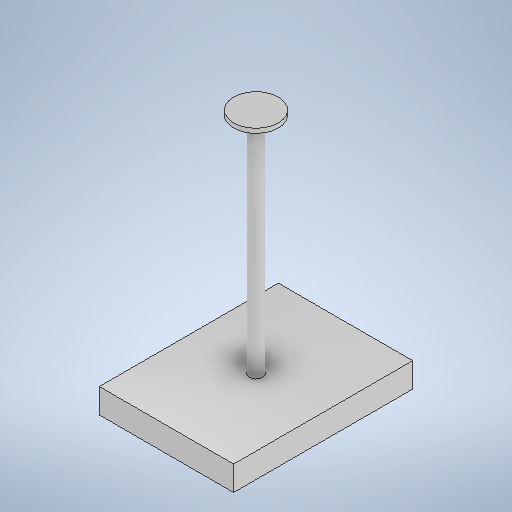
# Autodesk Inventor part: Corte
Saved by Autodesk Inventor 2025.2 (Build 292293000, 293)
## iProperties
Created: 2025-02-05
Part Number: Corte
Material: Generic
Document SubType Name: Modeling
Designer: Proyectos
Density: 1 g/cm^3
Appearance: Default
Author: Proyectos
Autodesk Inventor part; units mm, degrees
ref_plane "YZ Plane" through (0, 0, 0) normal (1, 0, 0) x (0, 1, 0)
ref_plane "XZ Plane" through (0, 0, 0) normal (0, 1, 0) x (-1, 0, 0)
ref_plane "XY Plane" through (0, 0, 0) normal (0, 0, 1) x (1, 0, 0)
sketch "Sketch1" plane through (0, 0, 0) normal (0, 1, 0) x (-1, 0, 0)
  line L0 (0, 0) -> (600, 0)
  line L1 (600, 0) -> (600, -800)
  line L2 (600, -800) -> (0, -800)
  line L3 (0, -800) -> (0, 0)
  line L4 (0, 0) -> (50, 0)
  line L5 (50, 0) -> (50, -50)
  line L6 (50, -50) -> (0, -50)
  line L7 (0, -50) -> (0, 0)
  line L8 (600, -800) -> (550, -800)
  line L9 (550, -800) -> (550, -750)
  line L10 (550, -750) -> (600, -750)
  line L11 (600, -750) -> (600, -800)
  line L12 (50, -50) -> (550, -50)
  line L13 (550, -50) -> (550, -750)
  line L14 (550, -750) -> (50, -750)
  line L15 (50, -750) -> (50, -50)
  dimension "d0" = 800
  dimension "d1" = 600
  dimension "d2" = 50
  dimension "d3" = 50
  dimension "d4" = 50
  dimension "d5" = 50
  constraints: 32 end point, 8 parallel, 4 horizontal, 4 perpendicular
  measures "d0" distance of L0.end L1.end
  measures "d1" distance of L1.end L2.end
  measures "d2" distance of L5.end L6.end
  measures "d3" distance of L4.end L5.end
  measures "d4" distance of L9.end L10.end
  measures "d5" distance of L8.end L9.end
extrude "Extrusion1" add sketch "Sketch1" along normal blind 100 contours L0 L5 L6 L3 | L0 L1 L10 L13 L12 L5 | L6 L15 L14 L9 L2 L3 | L1 L2 L9 L10
sketch "Sketch2" plane through (0, 100, 0) normal (0, 1, 0) x (1, 0, 0)
  line L0 (-600, 800) -> (-600, 0) projected
  line L1 (0, 0) -> (0, 800) projected
  line L2 (-600, 0) -> (0, 0)
  line L3 (0, 0) -> (0, 800)
  line L4 (0, 800) -> (-600, 800)
  line L5 (-600, 800) -> (-600, 0)
  circle A0 centre (-300, 400) radius 25
  dimension "d8" = 50
  constraints: 8 end point, 2 parallel, 1 centre point, 1 horizontal, 1 perpendicular
  measures "d8" diameter of A0
extrude "Extrusion2" add sketch "Sketch2" along normal blind 10 contours L4 L1 L2 L0 | A0
sketch "Sketch3" plane through (0, 110, 0) normal (0, 1, 0) x (1, 0, 0)
  line L0 (0, 0) -> (0, 800) projected
  line L1 (0, 800) -> (-600, 800) projected
  line L2 (-600, 800) -> (-600, 0) projected
  line L3 (-600, 0) -> (0, 0) projected
  circle A0 centre (-300, 400) radius 30
  dimension "d11" = 60
  constraints: 1 centre point
  measures "d11" diameter of A0
extrude "Extrusion3" add sketch "Sketch3" along normal blind 1000 contours A0
sketch "Sketch4" plane through (-300, 1110, -400) normal (0, 1, 0) x (1, 0, 0)
  circle A0 centre (0, 0) radius 30 projected
  circle A1 centre (0, 0) radius 100
  point P0 (300, -400)
  dimension "d14" = 200
  constraints: 1 centre point, 1 coincident
  measures "d14" diameter of A1
extrude "Extrusion4" add sketch "Sketch4" along normal blind 20 contours A0 | A1
body "Solid1"
